Autodesk Fusion 360 part; units mm, degrees
(part 4 of 4)
  line L3219 (-15, -90.7321) -> (-14, -90.7321)
  line L3220 (-23, -90.7321) -> (-22.5, -89.866)
  line L3221 (-27, -89) -> (-27.5, -89.866)
  line L3222 (-23, -89) -> (-24, -89)
  line L3223 (-42, -90.7321) -> (-41, -90.7321)
  line L3224 (-48, -90.7321) -> (-47, -90.7321)
  line L3225 (-27, -90.7321) -> (-26, -90.7321)
  line L3226 (-47, -90.7321) -> (-46.5, -89.866)
  line L3227 (-47, -89) -> (-48, -89)
  line L3228 (-26, -89) -> (-27, -89)
  line L3229 (-48, -89) -> (-48.5, -89.866)
  line L3230 (-27.5, -89.866) -> (-27, -90.7321)
  line L3231 (-21, -89) -> (-21.5, -89.866)
  line L3232 (-19.5, -89.866) -> (-20, -89)
  line L3233 (-22.5, -89.866) -> (-23, -89)
  line L3234 (-26, -90.7321) -> (-25.5, -89.866)
  line L3235 (-25.5, -89.866) -> (-26, -89)
  line L3236 (-24, -89) -> (-24.5, -89.866)
  line L3237 (-45.5, -89.866) -> (-45, -90.7321)
  line L3238 (-21, -90.7321) -> (-20, -90.7321)
  line L3239 (-24.5, -89.866) -> (-24, -90.7321)
  line L3240 (-48.5, -89.866) -> (-48, -90.7321)
  line L3241 (-20, -90.7321) -> (-19.5, -89.866)
  line L3242 (-24, -90.7321) -> (-23, -90.7321)
  line L3243 (-14, -89) -> (-15, -89)
  point P0 (-68.5, -11.866)
  point P1 (-62.5, -11.866)
  point P2 (-56.5, -11.866)
  point P3 (-50.5, -11.866)
  point P4 (-44.5, -11.866)
  point P5 (-38.5, -11.866)
  point P6 (-32.5, -11.866)
  point P7 (-26.5, -11.866)
  point P8 (-20.5, -11.866)
  point P9 (-14.5, -11.866)
  point P10 (-68.5, -14.866)
  point P11 (-62.5, -14.866)
  point P12 (-56.5, -14.866)
  point P13 (-50.5, -14.866)
  point P14 (-44.5, -14.866)
  point P15 (-38.5, -14.866)
  point P16 (-26.5, -14.866)
  point P17 (-32.5, -14.866)
  point P18 (-20.5, -14.866)
  point P19 (-14.5, -14.866)
  point P20 (-68.5, -17.866)
  point P21 (-62.5, -20.866)
  point P22 (-44.5, -20.866)
  point P23 (-56.5, -20.866)
  point P24 (-50.5, -20.866)
  point P25 (-20.5, -20.866)
  point P26 (-32.5, -20.866)
  point P27 (-38.5, -20.866)
  point P28 (-26.5, -20.866)
  point P29 (-14.5, -20.866)
  point P30 (-62.5, -17.866)
  point P31 (-56.5, -17.866)
  point P32 (-50.5, -17.866)
  point P33 (-44.5, -17.866)
  point P34 (-38.5, -17.866)
  point P35 (-26.5, -17.866)
  point P36 (-32.5, -17.866)
  point P37 (-20.5, -17.866)
  point P38 (-14.5, -17.866)
  point P39 (-68.5, -20.866)
  point P40 (-68.5, -23.866)
  point P41 (-62.5, -26.866)
  point P42 (-44.5, -26.866)
  point P43 (-56.5, -26.866)
  point P44 (-50.5, -26.866)
  point P45 (-20.5, -26.866)
  point P46 (-32.5, -26.866)
  point P47 (-38.5, -26.866)
  point P48 (-26.5, -26.866)
  point P49 (-14.5, -26.866)
  point P50 (-44.5, -32.866)
  point P51 (-62.5, -32.866)
  point P52 (-56.5, -32.866)
  point P53 (-68.5, -29.866)
  point P54 (-50.5, -32.866)
  point P55 (-32.5, -32.866)
  point P56 (-38.5, -32.866)
  point P57 (-20.5, -32.866)
  point P58 (-26.5, -32.866)
  point P59 (-14.5, -32.866)
  point P60 (-62.5, -29.866)
  point P61 (-56.5, -29.866)
  point P62 (-50.5, -29.866)
  point P63 (-44.5, -29.866)
  point P64 (-20.5, -29.866)
  point P65 (-26.5, -29.866)
  point P66 (-38.5, -29.866)
  point P67 (-32.5, -29.866)
  point P68 (-68.5, -32.866)
  point P69 (-14.5, -29.866)
  point P70 (-62.5, -23.866)
  point P71 (-56.5, -23.866)
  point P72 (-50.5, -23.866)
  point P73 (-44.5, -23.866)
  point P74 (-38.5, -23.866)
  point P75 (-26.5, -23.866)
  point P76 (-32.5, -23.866)
  point P77 (-20.5, -23.866)
  point P78 (-14.5, -23.866)
  point P79 (-68.5, -26.866)
  point P80 (-68.5, -35.866)
  point P81 (-62.5, -38.866)
  point P82 (-44.5, -38.866)
  point P83 (-56.5, -38.866)
  point P84 (-50.5, -38.866)
  point P85 (-20.5, -38.866)
  point P86 (-32.5, -38.866)
  point P87 (-38.5, -38.866)
  point P88 (-26.5, -38.866)
  point P89 (-14.5, -38.866)
  point P90 (-44.5, -44.866)
  point P91 (-62.5, -44.866)
  point P92 (-56.5, -44.866)
  point P93 (-68.5, -41.866)
  point P94 (-50.5, -44.866)
  point P95 (-32.5, -44.866)
  point P96 (-38.5, -44.866)
  point P97 (-20.5, -44.866)
  point P98 (-26.5, -44.866)
  point P99 (-14.5, -44.866)
  point P100 (-62.5, -41.866)
  point P101 (-56.5, -41.866)
  point P102 (-50.5, -41.866)
  point P103 (-44.5, -41.866)
  point P104 (-62.5, -53.866)
  point P105 (-14.5, -56.866)
  point P106 (-56.5, -53.866)
  point P107 (-50.5, -53.866)
  point P108 (-26.5, -53.866)
  point P109 (-44.5, -53.866)
  point P110 (-38.5, -53.866)
  point P111 (-20.5, -53.866)
  point P112 (-32.5, -53.866)
  point P113 (-68.5, -56.866)
  point P114 (-62.5, -47.866)
  point P115 (-14.5, -53.866)
  point P116 (-56.5, -47.866)
  point P117 (-50.5, -47.866)
  point P118 (-26.5, -47.866)
  point P119 (-38.5, -47.866)
  point P120 (-44.5, -47.866)
  point P121 (-20.5, -47.866)
  point P122 (-32.5, -47.866)
  point P123 (-14.5, -47.866)
  point P124 (-68.5, -50.866)
  point P125 (-20.5, -41.866)
  point P126 (-26.5, -41.866)
  point P127 (-38.5, -41.866)
  point P128 (-32.5, -41.866)
  point P129 (-68.5, -44.866)
  point P130 (-14.5, -41.866)
  point P131 (-68.5, -47.866)
  point P132 (-62.5, -50.866)
  point P133 (-50.5, -50.866)
  point P134 (-44.5, -50.866)
  point P135 (-56.5, -50.866)
  point P136 (-32.5, -50.866)
  point P137 (-20.5, -50.866)
  point P138 (-26.5, -50.866)
  point P139 (-38.5, -50.866)
  point P140 (-14.5, -50.866)
  point P141 (-44.5, -56.866)
  point P142 (-68.5, -53.866)
  point P143 (-50.5, -56.866)
  point P144 (-62.5, -56.866)
  point P145 (-56.5, -56.866)
  point P146 (-32.5, -56.866)
  point P147 (-38.5, -56.866)
  point P148 (-26.5, -56.866)
  point P149 (-20.5, -56.866)
  point P150 (-62.5, -35.866)
  point P151 (-56.5, -35.866)
  point P152 (-50.5, -35.866)
  point P153 (-44.5, -35.866)
  point P154 (-38.5, -35.866)
  point P155 (-26.5, -35.866)
  point P156 (-32.5, -35.866)
  point P157 (-20.5, -35.866)
  point P158 (-14.5, -35.866)
  point P159 (-68.5, -38.866)
  point P160 (-14.5, -59.866)
  point P161 (-68.5, -62.866)
  point P162 (-68.5, -65.866)
  point P163 (-62.5, -68.866)
  point P164 (-50.5, -68.866)
  point P165 (-44.5, -68.866)
  point P166 (-32.5, -68.866)
  point P167 (-56.5, -68.866)
  point P168 (-20.5, -68.866)
  point P169 (-26.5, -68.866)
  point P170 (-38.5, -68.866)
  point P171 (-68.5, -71.866)
  point P172 (-44.5, -74.866)
  point P173 (-50.5, -74.866)
  point P174 (-14.5, -68.866)
  point P175 (-62.5, -74.866)
  point P176 (-56.5, -74.866)
  point P177 (-32.5, -74.866)
  point P178 (-38.5, -74.866)
  point P179 (-26.5, -74.866)
  point P180 (-20.5, -74.866)
  point P181 (-56.5, -71.866)
  point P182 (-14.5, -74.866)
  point P183 (-50.5, -71.866)
  point P184 (-44.5, -71.866)
  point P185 (-26.5, -71.866)
  point P186 (-20.5, -71.866)
  point P187 (-38.5, -71.866)
  point P188 (-32.5, -71.866)
  point P189 (-68.5, -74.866)
  point P190 (-62.5, -65.866)
  point P191 (-50.5, -65.866)
  point P192 (-56.5, -65.866)
  point P193 (-14.5, -71.866)
  point P194 (-26.5, -65.866)
  point P195 (-38.5, -65.866)
  point P196 (-44.5, -65.866)
  point P197 (-20.5, -65.866)
  point P198 (-32.5, -65.866)
  point P199 (-14.5, -65.866)
  point P200 (-38.5, -59.866)
  point P201 (-20.5, -59.866)
  point P202 (-68.5, -68.866)
  point P203 (-26.5, -59.866)
  point P204 (-32.5, -59.866)
  point P205 (-50.5, -59.866)
  point P206 (-44.5, -59.866)
  point P207 (-62.5, -71.866)
  point P208 (-44.5, -62.866)
  point P209 (-62.5, -62.866)
  point P210 (-68.5, -59.866)
  point P211 (-50.5, -62.866)
  point P212 (-56.5, -62.866)
  point P213 (-38.5, -62.866)
  point P214 (-32.5, -62.866)
  point P215 (-20.5, -62.866)
  point P216 (-62.5, -59.866)
  point P217 (-26.5, -62.866)
  point P218 (-14.5, -62.866)
  point P219 (-56.5, -59.866)
  point P220 (-50.5, -80.866)
  point P221 (-68.5, -77.866)
  point P222 (-44.5, -80.866)
  point P223 (-62.5, -80.866)
  point P224 (-56.5, -80.866)
  point P225 (-32.5, -80.866)
  point P226 (-38.5, -80.866)
  point P227 (-14.5, -80.866)
  point P228 (-26.5, -80.866)
  point P229 (-20.5, -80.866)
  point P230 (-56.5, -77.866)
  point P231 (-50.5, -77.866)
  point P232 (-26.5, -77.866)
  point P233 (-44.5, -77.866)
  point P234 (-20.5, -77.866)
  point P235 (-38.5, -77.866)
  point P236 (-32.5, -77.866)
  point P237 (-68.5, -80.866)
  point P238 (-14.5, -77.866)
  point P239 (-62.5, -77.866)
  point P240 (-56.5, -86.866)
  point P241 (-62.5, -86.866)
  point P242 (-32.5, -86.866)
  point P243 (-50.5, -86.866)
  point P244 (-68.5, -83.866)
  point P245 (-44.5, -86.866)
  point P246 (-38.5, -86.866)
  point P247 (-26.5, -86.866)
  point P248 (-20.5, -86.866)
  point P249 (-14.5, -86.866)
  point P250 (-56.5, -83.866)
  point P251 (-26.5, -83.866)
  point P252 (-44.5, -83.866)
  point P253 (-50.5, -83.866)
  point P254 (-20.5, -83.866)
  point P255 (-38.5, -83.866)
  point P256 (-14.5, -83.866)
  point P257 (-32.5, -83.866)
  point P258 (-68.5, -86.866)
  point P259 (-62.5, -83.866)
  point P260 (-68.5, -89.866)
  point P261 (-62.5, -89.866)
  point P262 (-32.5, -89.866)
  point P263 (-56.5, -89.866)
  point P264 (-44.5, -89.866)
  point P265 (-38.5, -89.866)
  point P266 (-26.5, -89.866)
  point P267 (-20.5, -89.866)
  point P268 (-50.5, -89.866)
  point P269 (-14.5, -89.866)
extrude "Extrude11" cut sketch "Sketch7" against normal blind 5 contours L3 L3154 L3157 L3162 | L3 L3149 L3154 L3162 L3164 L3167 | L3 L3159 L3169 L3219 | L3 L3153 L3159 L3163 L3169 L3243 | L3 L3133 L3134 L3141 L3144 L3204 | L3 L3133 L3141 L3202 | L3 L3151 L3161 L3166 | L3 L3148 L3151 L3155 L3158 L3161 | L3 L3138 L3143 L3196 L3197 L3198 | L3 L3135 L3138 L3197 | L3 L3217 L3238 L3241 | L3 L3217 L3218 L3231 L3232 L3241 | L3 L3128 L3207 L3209 L3212 L3213 | L3 L3128 L3207 L3215 | L3 L3220 L3239 L3242 | L3 L3220 L3222 L3233 L3236 L3239 | L3 L3124 L3130 L3210 L3214 L3216 | L3 L3124 L3126 L3130 | L3 L3225 L3230 L3234 | L3 L3221 L3228 L3230 L3234 L3235 | L3 L3125 L3129 L3206 L3208 L3211 | L3 L3125 L3129 L3139 | L3 L3171 L3179 L3181 | L3 L3175 L3179 L3181 L3187 L3194 | L3 L3127 L3136 L3142 L3200 L3205 | L3 L3136 L3142 L3203 | L3 L3178 L3190 L3192 | L3 L3174 L3177 L3184 L3190 L3192 | L3 L3131 L3137 L3140 L3195 L3201 | L3 L3132 L3140 L3201 | L3 L3176 L3180 L3193 | L3 L3173 L3176 L3182 L3185 L3193 | L3 L3199 L3226 L3227 L3229 L3240 | L3 L3224 L3226 L3240 | L3 L3170 L3183 L3186 | L3 L3170 L3172 L3183 L3188 L3189 | L3 L3147 L3150 L3168 L3191 L3237 | L3 L3165 L3168 L3237 | L3 L3152 L3160 L3223 | L3 L3145 L3146 L3152 L3156 L3160 | L4 L5 L6 L7 L8 L9 | L10 L11 L12 L13 L14 L15 | L16 L17 L22 L24 L26 L27 | L18 L19 L20 L21 L23 L25 | L28 L29 L36 L38 L41 L48 | L30 L31 L37 L39 L50 L51 | L32 L34 L35 L42 L46 L47 | L33 L40 L43 L44 L45 L49 | L52 L54 L57 L94 L96 L98 | L53 L63 L72 L85 L95 L99 | L55 L60 L64 L70 L71 L73 | L56 L62 L66 L90 L92 L93 | L58 L76 L77 L79 L80 L91 | L59 L75 L82 L84 L88 L89 | L61 L65 L67 L68 L69 L97 | L74 L78 L81 L83 L86 L87 | L100 L102 L103 L106 L107 L111 | L101 L104 L105 L108 L109 L110 | L112 L113 L114 L117 L120 L123 | L115 L116 L118 L119 L121 L122 | L124 L137 L138 L140 L183 L238 | L125 L200 L202 L204 L213 L218 | L126 L134 L214 L217 L221 L225 | L127 L128 L130 L192 L216 L235 | L129 L195 L209 L211 L230 L234 | L131 L190 L197 L198 L212 L227 | L132 L136 L193 L206 L224 L226 | L133 L187 L203 L205 L219 L222 | L135 L188 L189 L208 L223 L233 | L139 L142 L144 L177 L180 L241 | L141 L149 L151 L174 L182 L185 | L143 L145 L172 L184 L242 L243 | L146 L154 L157 L162 L167 L170 | L147 L148 L150 L153 L161 L169 | L152 L155 L173 L179 L181 L237 | L156 L158 L163 L164 L166 L231 | L159 L160 L165 L168 L171 L228 | L175 L176 L178 L186 L239 L240 | L191 L194 L196 L199 L207 L229 | L201 L210 L215 L220 L232 L236 | L244 L246 L250 L426 L428 L439 | L245 L247 L254 L262 L315 L415 | L248 L259 L261 L413 L417 L421 | L249 L251 L252 L255 L311 L414 | L253 L307 L308 L416 L423 L424 | L256 L257 L429 L430 L435 L436 | L258 L304 L419 L422 L431 L438 | L260 L316 L412 L432 L433 L437 | L263 L265 L280 L286 L295 L296 | L264 L276 L302 L447 L474 L476 | L266 L272 L275 L277 L288 L298 | L267 L273 L440 L443 L446 L483 | L268 L283 L297 L442 L467 L473 | L269 L270 L282 L287 L293 L303 | L271 L289 L479 L480 L481 L482 | L274 L279 L291 L292 L299 L301 | L278 L281 L284 L300 L441 L475 | L285 L290 L294 L444 L456 L478 | L305 L310 L313 L314 L420 L427 | L306 L309 L312 L418 L425 L434 | L317 L321 L326 L331 L397 L398 | L318 L319 L330 L391 L392 L406 | L320 L375 L377 L384 L388 L410 | L322 L329 L332 L389 L395 L407 | L323 L327 L328 L376 L385 L396 | L324 L325 L374 L386 L387 L390 | L333 L343 L352 L358 L365 L470 | L334 L344 L369 L383 L394 L399 | L335 L348 L351 L357 L381 L411 | L336 L337 L342 L359 L380 L393 | L338 L347 L368 L382 L401 L408 | L339 L346 L355 L370 L371 L378 | L340 L350 L353 L366 L372 L404 | L341 L373 L445 L448 L449 L477 | L345 L356 L361 L364 L465 L468 | L349 L367 L402 L403 L405 L472 | L354 L362 L363 L379 L400 L409 | L360 L450 L451 L454 L461 L469 | L452 L459 L460 L462 L463 L471 | L453 L455 L457 L458 L464 L466 | L484 L497 L502 L503 L953 L955 | L485 L489 L490 L494 L496 L505 | L486 L493 L499 L500 L508 L952 | L487 L491 L498 L504 L507 L960 | L488 L495 L506 L961 L962 L963 | L492 L501 L951 L957 L958 L959 | L509 L831 L833 L836 L861 L864 | L510 L512 L767 L773 L775 L863 | L511 L513 L772 L832 L837 L956 | L514 L515 L517 L768 L774 L835 | L516 L765 L766 L769 L770 L954 | L518 L771 L830 L834 L860 L862 | L519 L526 L540 L554 L561 L704 | L520 L528 L578 L589 L590 L600 | L521 L531 L538 L545 L547 L568 | L522 L539 L552 L574 L579 L594 | L523 L542 L543 L548 L690 L694 | L524 L534 L553 L557 L569 L570 | L525 L527 L537 L549 L551 L563 | L529 L530 L535 L550 L556 L572 | L532 L533 L677 L682 L696 L699 | L536 L571 L585 L586 L587 L593 | L541 L546 L678 L688 L697 L700 | L544 L558 L559 L562 L675 L684 | L555 L564 L575 L576 L601 L602 | L560 L673 L681 L691 L698 L702 | L565 L685 L693 L695 L703 L706 | L566 L591 L592 L808 L816 L820 | L567 L573 L793 L809 L818 L825 | L577 L595 L599 L819 L826 L827 | L580 L596 L790 L794 L798 L807 | L581 L604 L792 L804 L805 L828 | L582 L605 L800 L803 L821 L829 | L583 L796 L813 L815 L817 L823 | L584 L588 L598 L802 L812 L814 | L597 L603 L795 L799 L806 L810 | L606 L635 L662 L663 L668 L672 | L607 L617 L634 L648 L667 L670 | L608 L679 L721 L730 L735 L742 | L609 L613 L615 L618 L641 L652 | L610 L612 L627 L644 L650 L657 | L611 L616 L623 L640 L727 L736 | L614 L633 L649 L651 L669 L671 | L619 L626 L716 L717 L731 L741 | L620 L624 L625 L653 L654 L661 | L621 L630 L631 L642 L665 L666 | L622 L637 L639 L647 L659 L660 | L628 L636 L646 L655 L656 L664 | L629 L632 L638 L643 L645 L658 | L674 L689 L701 L733 L737 L738 | L676 L680 L686 L687 L692 L705 | L683 L708 L723 L725 L728 L734 | L707 L711 L712 L713 L722 L724 | L709 L710 L718 L719 L720 L729 | L714 L715 L726 L732 L739 L740 | L743 L745 L762 L873 L875 L914 | L744 L748 L751 L753 L760 L878 | L746 L752 L754 L755 L764 L882 | L747 L750 L759 L763 L879 L880 | L749 L756 L757 L758 L877 L883 | L761 L874 L876 L881 L884 L885 | L776 L781 L783 L789 L845 L856 | L777 L787 L838 L849 L857 L858 | L778 L779 L786 L840 L848 L853 | L780 L784 L839 L844 L851 L855 | L782 L785 L788 L841 L852 L854 | L791 L797 L801 L811 L822 L824 | L842 L843 L846 L847 L850 L859 | L865 L866 L871 L918 L925 L949 | L867 L869 L894 L898 L904 L938 | L868 L888 L902 L910 L912 L923 | L870 L908 L909 L913 L934 L942 | L872 L886 L903 L919 L922 L926 | L887 L890 L899 L900 L901 L916 | L889 L915 L930 L944 L946 L947 | L891 L897 L921 L931 L940 L950 | L892 L924 L928 L936 L943 L945 | L893 L895 L905 L920 L935 L939 | L896 L907 L911 L917 L937 L941 | L906 L927 L929 L932 L933 L948 | L964 L978 L1056 L1066 L1714 L1724 | L965 L997 L999 L1005 L1719 L1725 | L966 L967 L972 L990 L1004 L1734 | L968 L998 L1007 L1040 L1063 L1732 | L969 L995 L1002 L1006 L1047 L1740 | L970 L979 L985 L1001 L1043 L1074 | L971 L975 L980 L1721 L1723 L1730 | L973 L981 L983 L984 L989 L992 | L974 L982 L991 L1713 L1715 L1735 | L976 L1000 L1044 L1048 L1050 L1731 | L977 L987 L988 L1736 L1737 L1738 | L986 L993 L994 L996 L1003 L1712 | L1008 L1012 L1016 L1070 L1781 L1792 | L1009 L1013 L1017 L1026 L1029 L1090 | L1010 L1019 L1028 L1079 L1083 L1085 | L1011 L1021 L1023 L1031 L1062 L1089 | L1014 L1015 L1024 L1071 L1076 L1086 | L1018 L1381 L1405 L1410 L1779 L1914 | L1020 L1776 L1778 L1793 L1798 L1804 | L1022 L1058 L1068 L1077 L1084 L1091 | L1025 L1033 L1037 L1059 L1780 L1797 | L1027 L1032 L1036 L1054 L1787 L1795 | L1030 L1061 L1069 L1081 L1087 L1088 | L1034 L1035 L1064 L1067 L1072 L1080 | L1038 L1039 L1046 L1052 L1075 L1078 | L1041 L1042 L1045 L1053 L1057 L1065 | L1049 L1051 L1055 L1060 L1073 L1082 | L1092 L1106 L1116 L1119 L1624 L1625 | L1093 L1095 L1109 L1110 L1629 L1649 | L1094 L1103 L1120 L1135 L1136 L1655 | L1096 L1097 L1125 L1129 L1131 L1636 | L1098 L1122 L1677 L1812 L1818 L1838 | L1099 L1651 L1675 L1680 L1816 L1831 | L1100 L1114 L1657 L1659 L1661 L1690 | L1101 L1126 L1138 L1660 L1664 L1689 | L1102 L1112 L1113 L1128 L1623 L1694 | L1104 L1672 L1678 L1692 L1829 L1851 | L1105 L1665 L1666 L1667 L1691 L1693 | L1107 L1142 L1152 L1616 L1646 L1648 | L1108 L1123 L1124 L1130 L1132 L1634 | L1111 L1153 L1569 L1627 L1641 L1647 | L1115 L1117 L1121 L1622 L1628 L1638 | L1118 L1127 L1133 L1134 L1615 L1626 | L1137 L1618 L1630 L1642 L1643 L1644 | L1139 L1140 L1570 L1590 L1607 L1609 | L1141 L1147 L1171 L1189 L1190 L1704 | L1143 L1162 L1586 L1600 L1603 L1613 | L1144 L1149 L1154 L1158 L1163 L1611 | L1145 L1150 L1175 L1178 L1181 L1697 | L1146 L1608 L1621 L1633 L1635 L1637 | L1148 L1157 L1160 L1165 L1166 L1606 | L1151 L1156 L1167 L1173 L1182 L1574 | L1155 L1177 L1179 L1421 L1426 L1707 | L1159 L1161 L1164 L1573 L1610 L1612 | L1168 L1170 L1174 L1176 L1695 L1764 | L1169 L1184 L1185 L1593 L1595 L1602 | L1172 L1180 L1428 L1699 L1766 L1768 | L1183 L1187 L1188 L1696 L1703 L1767 | L1186 L1418 L1427 L1706 L1717 L1765 | L1191 L1742 L1751 L1756 L1762 L1808 | L1192 L1194 L1196 L1198 L1837 L1846 | L1193 L1197 L1200 L1204 L1747 L1760 | L1195 L1202 L1211 L1219 L1819 L1849 | L1199 L1218 L1811 L1815 L1824 L1841 | L1201 L1208 L1212 L1749 L1755 L1761 | L1203 L1206 L1753 L1757 L1758 L1807 | L1205 L1210 L1215 L1217 L1839 L1847 | L1207 L1216 L1743 L1748 L1752 L1754 | L1209 L1822 L1832 L1840 L1842 L1845 | L1213 L1214 L1825 L1843 L1850 L1853 | L1220 L1224 L1262 L1275 L1295 L1296 | L1221 L1260 L1269 L1272 L1293 L1314 | L1222 L1249 L1279 L1280 L1294 L1502 | L1223 L1231 L1281 L1298 L1509 L1527 | L1225 L1273 L1282 L1288 L1516 L1541 | L1226 L1263 L1265 L1289 L1300 L1534 | L1227 L1242 L1245 L1255 L1256 L1285 | L1228 L1248 L1310 L1321 L1325 L1532 | L1229 L1236 L1243 L1286 L1311 L1317 | L1230 L1241 L1254 L1270 L1292 L1526 | L1232 L1246 L1274 L1287 L1290 L1506 | L1233 L1240 L1251 L1253 L1539 L1540 | L1234 L1244 L1258 L1283 L1291 L1316 | L1235 L1250 L1259 L1261 L1266 L1276 | L1237 L1257 L1268 L1320 L1336 L1504 | L1238 L1252 L1267 L1297 L1522 L1531 | L1239 L1318 L1332 L1342 L1346 L1347 | L1247 L1308 L1309 L1315 L1326 L1329 | L1264 L1271 L1278 L1299 L1305 L1306 | L1277 L1284 L1313 L1338 L1341 L1343 | L1301 L1327 L1353 L1435 L1438 L1455 | L1302 L1359 L1362 L1366 L1368 L1451 | L1303 L1304 L1340 L1344 L1367 L1372 | L1307 L1337 L1349 L1364 L1450 L1462 | L1312 L1322 L1323 L1330 L1331 L1335 | L1319 L1324 L1333 L1339 L1348 L1373 | L1328 L1334 L1352 L1360 L1361 L1371 | L1345 L1356 L1369 L1432 L1440 L1463 | L1350 L1354 L1355 L1363 L1444 L1466 | L1351 L1358 L1365 L1436 L1447 L1467 | L1357 L1437 L1458 L1460 L1461 L1468 | L1370 L1434 L1439 L1445 L1453 L1454 | L1374 L1376 L1441 L1456 L1464 L1465 | L1375 L1443 L1448 L1452 L1457 L1459 | L1377 L1379 L1400 L1414 L1788 L1796 | L1378 L1382 L1383 L1384 L1413 L1900 | L1380 L1392 L1401 L1407 L1412 L1901 | L1385 L1398 L1406 L1905 L1906 L1918 | L1386 L1391 L1393 L1395 L1404 L1416 | L1387 L1397 L1408 L1409 L1904 L1921 | L1388 L1389 L1415 L1899 L1919 L1922 | L1390 L1402 L1783 L1791 L1794 L1803 | L1394 L1396 L1782 L1790 L1800 L1801 | L1399 L1770 L1771 L1775 L1786 L1805 | L1403 L1411 L1769 L1773 L1774 L1785 | L1417 L1705 L1710 L1716 L1733 L1741 | L1419 L1422 L1700 L1709 L1711 L1729 | L1420 L1429 L1430 L1718 L1722 L1763 | L1423 L1698 L1701 L1720 L1726 L1739 | L1424 L1425 L1702 L1708 L1727 L1728 | L1431 L1446 L1477 L1484 L1493 L1498 | L1433 L1479 L1488 L1490 L1497 L1500 | L1442 L1496 L1866 L1879 L1885 L1888 | L1449 L1474 L1476 L1478 L1483 L1494 | L1469 L1482 L1865 L1874 L1882 L1913 | L1470 L1475 L1486 L1495 L1856 L1890 | L1471 L1481 L1860 L1870 L1896 L1911 | L1472 L1491 L1871 L1883 L1891 L1909 | L1473 L1489 L1855 L1863 L1881 L1892 | L1480 L1487 L1861 L1862 L1895 L1923 | L1485 L1499 L1869 L1884 L1886 L1887 | L1492 L1872 L1878 L1889 L1903 L1908 | L1501 L1517 L1524 L1525 L1549 L1554 | L1503 L1520 L1542 L1557 L1562 L1567 | L1505 L1529 L1536 L1538 L1558 L1561 | L1507 L1530 L1537 L1544 L1547 L1551 | L1508 L1533 L1546 L1552 L1564 L1565 | L1510 L1515 L1523 L1555 L1560 L1563 | L1511 L1512 L1513 L1535 L1545 L1566 | L1514 L1521 L1543 L1548 L1550 L1553 | L1518 L1519 L1528 L1556 L1559 L1568 | L1571 L1585 L1587 L1591 L1597 L1598 | L1572 L1575 L1577 L1579 L1631 L1650 | L1576 L1580 L1588 L1596 L1619 L1639 | L1578 L1581 L1584 L1589 L1592 L1640 | L1582 L1583 L1599 L1604 L1605 L1614 | L1594 L1601 L1617 L1620 L1632 L1645 | L1652 L1653 L1683 L1684 L1813 L1833 | L1654 L1676 L1817 L1823 L1827 L1835 | L1656 L1668 L1674 L1681 L1685 L1810 | L1658 L1673 L1821 L1826 L1834 L1852 | L1662 L1679 L1687 L1688 L1814 L1836 | L1663 L1820 L1828 L1830 L1844 L1848 | L1669 L1670 L1671 L1682 L1686 L1806 | L1744 L1745 L1746 L1750 L1759 L1809 | L1772 L1777 L1784 L1789 L1799 L1802 | L1854 L1864 L1867 L1868 L1880 L1897 | L1857 L1873 L1875 L1877 L1893 L1916 | L1858 L1859 L1876 L1894 L1910 L1912 | L1898 L1902 L1907 L1915 L1917 L1920 | L1924 L2272 L2275 L2634 L2640 L2642 | L1925 L1927 L2261 L2263 L2264 L2635 | L1926 L2266 L2268 L2270 L2638 L2639 | L1928 L1946 L1947 L1948 L1951 L1958 | L1929 L1935 L1939 L1944 L1952 L1961 | L1930 L1940 L1943 L2021 L2024 L2034 | L1931 L1942 L1950 L1955 L2014 L2036 | L1932 L1933 L1937 L2018 L2027 L2039 | L1934 L1949 L1954 L1964 L2022 L2038 | L1936 L1945 L1960 L1962 L1965 L1997 | L1938 L2011 L2013 L2019 L2031 L2032 | L1941 L2012 L2015 L2020 L2023 L2037 | L1953 L1956 L1957 L1959 L1963 L2001 | L1966 L1977 L1988 L1989 L2250 L2252 | L1967 L1980 L1984 L1986 L1995 L2002 | L1968 L2208 L2215 L2236 L2240 L2258 | L1969 L1970 L1976 L1982 L1985 L1987 | L1971 L1972 L1978 L1979 L1983 L1996 | L1973 L1991 L2511 L2516 L2577 L2598 | L1974 L1999 L2509 L2536 L2610 L2617 | L1975 L1981 L2552 L2558 L2597 L2614 | L1990 L2227 L2246 L2256 L2537 L2540 | L1992 L2204 L2211 L2248 L2251 L2253 | L1993 L1998 L2000 L2003 L2005 L2008 | L1994 L2004 L2006 L2007 L2009 L2010 | L2016 L2017 L2025 L2026 L2030 L2288 | L2028 L2029 L2033 L2035 L2279 L2283 | L2040 L2055 L2060 L2081 L2414 L2423 | L2041 L2045 L2048 L2062 L2419 L2620 | L2042 L2075 L2083 L2088 L2091 L2097 | L2043 L2046 L2047 L2054 L2066 L2068 | L2044 L2049 L2073 L2079 L2082 L2090 | L2050 L2052 L2056 L2059 L2412 L2484 | L2051 L2053 L2065 L2074 L2471 L2488 | L2057 L2061 L2063 L2086 L2434 L2459 | L2058 L2064 L2069 L2092 L2448 L2474 | L2067 L2071 L2084 L2085 L2094 L2099 | L2070 L2076 L2080 L2089 L2093 L2096 | L2072 L2077 L2078 L2087 L2095 L2098 | L2100 L2102 L2129 L2137 L2148 L2150 | L2101 L2104 L2115 L2149 L2151 L2154 | L2103 L2124 L2203 L2302 L2371 L2381 | L2105 L2110 L2118 L2142 L2144 L2153 | L2106 L2117 L2125 L2146 L2157 L2608 | L2107 L2120 L2122 L2133 L2143 L2147 | L2108 L2109 L2113 L2119 L2138 L2145 | L2111 L2127 L2317 L2332 L2384 L2397 | L2112 L2136 L2305 L2308 L2375 L2377 | L2114 L2123 L2126 L2132 L2152 L2156 | L2116 L2562 L2586 L2591 L2602 L2609 | L2121 L2588 L2596 L2605 L2613 L2615 | L2128 L2141 L2160 L2579 L2601 L2604 | L2130 L2134 L2139 L2140 L2155 L2158 | L2131 L2183 L2361 L2390 L2392 L2394 | L2135 L2161 L2165 L2166 L2184 L2191 | L2159 L2169 L2172 L2173 L2175 L2193 | L2162 L2170 L2350 L2354 L2383 L2395 | L2163 L2171 L2178 L2185 L2187 L2188 | L2164 L2174 L2176 L2180 L2182 L2186 | L2167 L2168 L2179 L2181 L2189 L2192 | L2177 L2190 L2337 L2352 L2368 L2370 | L2194 L2198 L2201 L2310 L2318 L2322 | L2195 L2197 L2298 L2301 L2309 L2323 | L2196 L2328 L2429 L2437 L2490 L2493 | L2199 L2303 L2306 L2311 L2325 L2330 | L2200 L2202 L2304 L2314 L2335 L2351 | L2205 L2206 L2574 L2590 L2594 L2599 | L2207 L2213 L2218 L2232 L2245 L2254 | L2209 L2231 L2521 L2544 L2548 L2553 | L2210 L2212 L2220 L2229 L2239 L2259 | L2214 L2223 L2238 L2241 L2244 L2255 | L2216 L2221 L2224 L2237 L2249 L2257 | L2217 L2507 L2512 L2513 L2534 L2547 | L2219 L2242 L2243 L2501 L2522 L2533 | L2222 L2228 L2518 L2542 L2546 L2554 | L2225 L2226 L2235 L2532 L2535 L2556 | L2230 L2233 L2524 L2569 L2593 L2611 | L2234 L2247 L2566 L2578 L2595 L2606 | L2260 L2267 L2273 L2274 L2637 L2641 | L2262 L2269 L2271 L2294 L2297 L2630 | L2265 L2286 L2290 L2627 L2636 L2643 | L2276 L2280 L2281 L2282 L2287 L2632 | L2277 L2284 L2291 L2295 L2623 L2628 | L2278 L2296 L2624 L2626 L2629 L2631 | L2285 L2289 L2292 L2293 L2625 L2633 | L2299 L2300 L2316 L2319 L2320 L2329 | L2307 L2362 L2420 L2440 L2476 L2494 | L2312 L2313 L2315 L2321 L2326 L2331 | L2324 L2327 L2402 L2411 L2426 L2497 | L2333 L2334 L2339 L2340 L2345 L2353 | L2336 L2338 L2355 L2374 L2380 L2388 | L2341 L2343 L2344 L2356 L2360 L2364 | L2342 L2346 L2359 L2366 L2369 L2387 | L2347 L2363 L2365 L2367 L2389 L2391 | L2348 L2349 L2433 L2457 L2485 L2489 | L2357 L2358 L2407 L2415 L2452 L2479 | L2372 L2378 L2379 L2385 L2393 L2396 | L2373 L2376 L2465 L2480 L2487 L2492 | L2382 L2398 L2399 L2403 L2428 L2432 | L2386 L2401 L2405 L2430 L2438 L2441 | L2400 L2404 L2406 L2431 L2435 L2436 | L2408 L2413 L2482 L2495 L2498 L2499 | L2409 L2417 L2425 L2619 L2621 L2622 | L2410 L2416 L2421 L2466 L2483 L2486 | L2418 L2422 L2424 L2444 L2464 L2478 | L2427 L2439 L2445 L2454 L2458 L2473 | L2442 L2447 L2455 L2468 L2469 L2477 | L2443 L2453 L2456 L2462 L2467 L2472 | L2446 L2450 L2460 L2461 L2470 L2475 | L2449 L2451 L2463 L2481 L2491 L2496 | L2500 L2503 L2573 L2581 L2582 L2583 | L2502 L2505 L2526 L2529 L2567 L2584 | L2504 L2517 L2519 L2520 L2527 L2565 | L2506 L2559 L2563 L2570 L2585 L2589 | L2508 L2514 L2525 L2530 L2545 L2549 | L2510 L2515 L2523 L2539 L2543 L2550 | L2528 L2564 L2568 L2575 L2580 L2587 | L2531 L2538 L2541 L2551 L2555 L2557 | L2560 L2561 L2571 L2592 L2603 L2616 | L2572 L2576 L2600 L2607 L2612 L2618 | L2644 L2645 L2683 L2684 L2685 L2702 | L2646 L2658 L2695 L2698 L2699 L2700 | L2647 L2649 L2682 L2692 L2838 L2875 | L2648 L2665 L2827 L2831 L2840 L2860 | L2650 L2664 L2688 L2691 L2854 L2857 | L2651 L2668 L2676 L2837 L2852 L2873 | L2652 L2653 L2667 L2678 L2686 L2690 | L2654 L2689 L2693 L2828 L2841 L2851 | L2655 L2671 L2674 L2679 L2687 L2872 | L2656 L2660 L2666 L2673 L2675 L2694 | L2657 L2669 L2672 L2681 L2849 L2874 | L2659 L2661 L2662 L2663 L2855 L2871 | L2670 L2680 L2696 L2697 L2703 L2706 | L2677 L2701 L2704 L2705 L2707 L2850 | L2708 L2775 L2795 L2797 L2876 L2881 | L2709 L2764 L2768 L2773 L2776 L2779 | L2710 L2772 L2799 L2801 L2803 L2879 | L2711 L2760 L2761 L2762 L2767 L2769 | L2712 L2777 L2781 L2809 L2811 L2813 | L2713 L2717 L2723 L2725 L2729 L2731 | L2714 L2719 L2722 L2726 L2728 L2736 | L2715 L2720 L2721 L2730 L2734 L2735 | L2716 L2718 L2724 L2727 L2732 L2733 | L2737 L2738 L2754 L2756 L2757 L2771 | L2739 L2742 L2745 L2746 L2751 L2752 | L2740 L2744 L2748 L2749 L2750 L2759 | L2741 L2743 L2747 L2753 L2755 L2758 | L2763 L2765 L2807 L2810 L2877 L2878 | L2766 L2778 L2782 L2880 L2882 L2883 | L2770 L2774 L2785 L2786 L2812 L2814 | L2780 L2796 L2798 L2804 L2806 L2808 | L2783 L2793 L2794 L2800 L2802 L2805 | L2784 L2787 L2789 L2829 L2836 L2861 | L2788 L2816 L2821 L2825 L2834 L2856 | L2790 L2791 L2792 L2817 L2822 L2832 | L2815 L2818 L2819 L2823 L2826 L2830 | L2820 L2833 L2835 L2843 L2844 L2862 | L2824 L2839 L2846 L2853 L2867 L2868 | L2842 L2848 L2858 L2865 L2866 L2869 | L2845 L2847 L2859 L2863 L2864 L2870 | L2884 L2886 L2889 L2893 L2920 L2946 | L2885 L2887 L2894 L2909 L2922 L2936 | L2888 L2890 L2892 L2907 L2910 L2952 | L2891 L2895 L2908 L2937 L2941 L2942 | L2896 L2898 L2902 L2904 L2905 L2916 | L2897 L2899 L2901 L2906 L2917 L3113 | L2900 L2903 L2913 L2914 L3099 L3109 | L2911 L2912 L2915 L3094 L3095 L3100 | L2918 L2928 L3008 L3012 L3017 L3018 | L2919 L2955 L2958 L2962 L2974 L2987 | L2921 L2929 L2931 L2938 L2940 L2943 | L2923 L2925 L2930 L2934 L2935 L2947 | L2924 L2933 L3003 L3019 L3020 L3021 | L2926 L2950 L2951 L2954 L2967 L2992 | L2927 L2932 L2975 L2994 L3011 L3016 | L2939 L2944 L2949 L2956 L2957 L2983 | L2945 L2966 L2970 L2977 L2981 L3006 | L2948 L2953 L2998 L3002 L3013 L3014 | L2959 L2960 L2969 L2993 L2996 L2997 | L2961 L2963 L2980 L2988 L2995 L3007 | L2964 L2965 L2968 L2979 L2990 L2991 | L2971 L2973 L2999 L3000 L3009 L3015 | L2972 L2982 L2984 L2986 L2989 L3004 | L2976 L2978 L2985 L3001 L3005 L3010 | L3022 L3033 L3038 L3114 L3122 L3123 | L3023 L3025 L3029 L3047 L3049 L3057 | L3024 L3037 L3052 L3053 L3065 L3119 | L3026 L3027 L3028 L3048 L3117 L3121 | L3030 L3034 L3035 L3061 L3116 L3120 | L3031 L3039 L3063 L3067 L3080 L3082 | L3032 L3040 L3062 L3066 L3072 L3086 | L3036 L3043 L3046 L3054 L3115 L3118 | L3041 L3044 L3064 L3074 L3081 L3101 | L3042 L3045 L3055 L3084 L3088 L3106 | L3050 L3056 L3083 L3087 L3096 L3112 | L3051 L3058 L3070 L3073 L3075 L3079 | L3059 L3069 L3076 L3077 L3078 L3110 | L3060 L3068 L3071 L3085 L3090 L3107 | L3089 L3092 L3098 L3102 L3105 L3111 | L3091 L3093 L3097 L3103 L3104 L3108 bodies 3
sketch "Sketch8" plane through (0, 24, 0) normal (0, -1, 0) x (1, 0, 0)
  line L0 (60.6044, -92.1931) -> (18.6044, -92.1931)
  line L1 (18.6044, -92.1931) -> (18.6044, -7.1931)
  line L2 (18.6044, -7.1931) -> (60.6044, -7.1931)
  line L3 (60.6044, -7.1931) -> (60.6044, -92.1931)
  line L4 (0, 0) -> (0, -100)
  line L5 (0, -100) -> (79, -100)
  line L6 (79, -100) -> (79, 0)
  line L7 (79, 0) -> (0, 0)
  line L8 (63, -91) -> (75, -91)
  line L9 (75, -91) -> (75, -9)
  line L10 (75, -9) -> (63, -9)
  line L11 (63, -9) -> (63, -91)
  line L12 (39.6044, -92.1931) -> (39.6044, -7.1931)
  line L13 (4.2088, -9) -> (16.2088, -9)
  line L14 (4.2088, -91) -> (4.2088, -9)
  line L15 (16.2088, -9) -> (16.2088, -91)
  line L16 (16.2088, -91) -> (4.2088, -91)
  constraint horizontal L8
  constraint vertical L9
  constraint horizontal L10
  constraint vertical L11
  constraint midpoint L0 L12.start
  constraint midpoint L2 L12.end
  constraint symmetric L8.start L12 L15.end
  constraint symmetric L8.end L12 L14.start
  constraint symmetric L9.end L12 L13.start
  constraint symmetric L10.end L12 L13.end
extrude "Extrude12" cut sketch "Sketch8" against normal blind 30 contours L8 L9 L10 L11 | L13 L14 L15 L16 bodies 3
sketch "Sketch9" plane through (0, 0, -100) normal (0, 0, 1) x (1, 0, 0)
  line L0 (0, 7) -> (79, 7)
  line L1 (79, 7) -> (79, 24)
  line L2 (79, 24) -> (0, 24)
  line L3 (0, 24) -> (0, 7)
  line L4 (1, 23) -> (78, 23)
  line L5 (78, 23) -> (78, 22)
  line L6 (78, 22) -> (1, 22)
  line L7 (1, 22) -> (1, 23)
  line L8 (1, 21) -> (78, 21)
  line L9 (78, 21) -> (78, 20)
  line L10 (78, 20) -> (1, 20)
  line L11 (1, 20) -> (1, 21)
  line L12 (1, 19) -> (78, 19)
  line L13 (78, 19) -> (78, 18)
  line L14 (78, 18) -> (1, 18)
  line L15 (1, 18) -> (1, 19)
  constraint horizontal L4
  constraint vertical L5
  constraint horizontal L6
  constraint vertical L7
  constraint horizontal L8
  constraint vertical L9
  constraint horizontal L10
  constraint vertical L11
  constraint horizontal L12
  constraint vertical L13
  constraint horizontal L14
  constraint vertical L15
extrude "Extrude13" cut sketch "Sketch9" against normal blind 26 contours L4 L5 L6 L7 | L8 L9 L10 L11 | L12 L13 L14 L15 bodies 3
sketch "Sketch10" plane through (0, 0, 0) normal (1, 0, 0) x (0, 0, -1)
  line L0 (0, 7) -> (100, 7)
  line L1 (100, 7) -> (100, 24)
  line L2 (100, 24) -> (0, 24)
  line L3 (0, 24) -> (0, 7)
  line L4 (1, 23) -> (99, 23)
  line L5 (99, 23) -> (99, 22)
  line L6 (99, 22) -> (1, 22)
  line L7 (1, 22) -> (1, 23)
  line L8 (1, 21) -> (99, 21)
  line L9 (99, 21) -> (99, 20)
  line L10 (99, 20) -> (1, 20)
  line L11 (1, 20) -> (1, 21)
  line L12 (1, 19) -> (99, 19)
  line L13 (99, 19) -> (99, 18)
  line L14 (99, 18) -> (1, 18)
  line L15 (1, 18) -> (1, 19)
  constraint horizontal L4
  constraint vertical L5
  constraint horizontal L6
  constraint vertical L7
  constraint horizontal L8
  constraint vertical L9
  constraint horizontal L10
  constraint vertical L11
  constraint horizontal L12
  constraint vertical L13
  constraint horizontal L14
  constraint vertical L15
extrude "Extrude14" cut sketch "Sketch10" against normal blind 29 contours L4 L5 L6 L7 | L8 L9 L10 L11 | L12 L13 L14 L15 bodies 3
extrude "Extrude15" cut sketch "Sketch9" along normal blind 126 contours L4 L5 L6 L7 | L8 L9 L10 L11 | L12 L13 L14 L15 bodies 3
extrude "Extrude16" cut sketch "Sketch10" along normal blind 112 contours L4 L5 L6 L7 | L8 L9 L10 L11 | L12 L13 L14 L15 bodies 3
move_body "Move3" bodies 1 to x (1, 0, 0) y (0, 1, 0) z (0, 0, 1) at (0, 4, 0)
extrude "Extrude17" cut 1 faces at (32.5348, 24, -97.3977) along direction (0, 1, 0) blind 4 on bodies 3 bodies 3
sketch "Sketch11" plane through (0, 0, 0) normal (1, 0, 0) x (0, 0, -1)
  line L0 (99, 23) -> (99, 22)
  line L1 (99, 22) -> (1, 22)
  line L2 (1, 22) -> (1, 23)
  line L3 (1, 23) -> (99, 23)
  line L4 (99, 21) -> (99, 20)
  line L5 (99, 20) -> (1, 20)
  line L6 (1, 20) -> (1, 21)
  line L7 (1, 21) -> (99, 21)
  line L8 (99, 19) -> (99, 18)
  line L9 (99, 18) -> (1, 18)
  line L10 (1, 18) -> (1, 19)
  line L11 (1, 19) -> (99, 19)
  line L12 (0, 7) -> (100, 7)
  line L13 (100, 7) -> (100, 28)
  line L14 (100, 28) -> (0, 28)
  line L15 (0, 28) -> (0, 7)
  line L16 (0, 17.5) -> (0.65, 17.5)
  line L17 (100, 17.5) -> (99.35, 17.5)
  line L18 (0.6563, 28.6) -> (100, 28.6)
  line L19 (100, 28.6) -> (100, 8.6)
  line L20 (100, 8.6) -> (0.6563, 8.6)
  line L21 (0.6563, 8.6) -> (0.6563, 28.6)
  line L22 (99.35, 28.6) -> (99.35, 8.6)
  dimension "d46" = 0.65
  dimension "d47" = 0.65
  constraint midpoint L15 L16.start
  constraint perpendicular L10 L16
  constraint midpoint L13 L17.start
  constraint perpendicular L13 L17
  constraint horizontal L18
  constraint vertical L19
  constraint horizontal L20
  constraint vertical L21
  constraint coincident L13 L19.end
  constraint coincident L18 L22.start
  constraint coincident L20 L22.end
  constraint perpendicular L20 L22
  measures "d46" distance of L16.start L16.end
  measures "d47" distance of L17.start L17.end
extrude "Extrude18" cut 1 faces at (32.5348, 28, -97.3977) along direction (0, 1, 0) blind 1 on bodies 3 bodies 3
extrude "Extrude19" cut sketch "Sketch11" against normal blind 18 contours L14 L20 L21 L22 | L14 L18 L21 L22 bodies 3
sketch "Sketch12" plane through (0, 0, 0) normal (0, 1, 0) x (1, 0, 0)
  line L0 (0, 100) -> (80, 100)
  line L1 (80, 100) -> (80, 0)
  line L2 (80, 0) -> (0, 0)
  line L3 (0, 0) -> (0, 100)
  constraint horizontal L0
  constraint vertical L1
  constraint horizontal L2
  constraint vertical L3
move_body "Move4" bodies 3 to x (1, 0, 0) y (0, 1, 0) z (0, 0, 1) at (0, -5.5, 0)
extrude "Extrude20" add sketch "Sketch12" along normal blind 1.6 separate body makes body 4
sketch "Sketch13" plane through (0, -47.8659, -38.2927) normal (0, -0.780869, -0.624695) x (-1, 0, 0)
  line L0 (-1, 104.6364) -> (-1, 103.0356)
  line L1 (-1, 103.0356) -> (-78, 103.0356)
  line L2 (-78, 103.0356) -> (-78, 104.6364)
  line L3 (-78, 104.6364) -> (-100, 104.6364)
  line L4 (-100, 104.6364) -> (-79, 77.7433)
  line L5 (-79, 77.7433) -> (-79, 79.0239)
  line L6 (-79, 79.0239) -> (0, 79.0239)
  line L7 (0, 79.0239) -> (20, 104.6364)
  line L8 (20, 104.6364) -> (-1, 104.6364)
  line L9 (-78, 96.6325) -> (-78, 98.2333)
  line L10 (-78, 98.2333) -> (-1, 98.2333)
  line L11 (-1, 98.2333) -> (-1, 96.6325)
  line L12 (-1, 96.6325) -> (-78, 96.6325)
  line L13 (-78, 99.8341) -> (-78, 101.4349)
  line L14 (-78, 101.4349) -> (-1, 101.4349)
  line L15 (-1, 101.4349) -> (-1, 99.8341)
  line L16 (-1, 99.8341) -> (-78, 99.8341)
  line L17 (-80, 85) -> (0, 85)
  line L18 (0, 85) -> (0, 79.1)
  line L19 (0, 79.1) -> (-80, 79.1)
  line L20 (-80, 79.1) -> (-80, 85)
  constraint horizontal L17
  constraint vertical L18
  constraint horizontal L19
  constraint vertical L20
extrude "Extrude21" add sketch "Sketch13" along normal blind 5 contours L17 L18 L19 L20 bodies 3
sketch "Sketch14" plane through (0, 0.9146, -0.7317) normal (0, -0.780869, 0.624695) x (1, 0, 0)
  line L0 (78, 26.5495) -> (78, 24.9488)
  line L1 (78, 24.9488) -> (1, 24.9488)
  line L2 (1, 24.9488) -> (1, 26.5495)
  line L3 (1, 26.5495) -> (-20, 26.5495)
  line L4 (-20, 26.5495) -> (0, 0.937)
  line L5 (0, 0.937) -> (79, 0.937)
  line L6 (79, 0.937) -> (79, -0.3436)
  line L7 (79, -0.3436) -> (100, 26.5495)
  line L8 (100, 26.5495) -> (78, 26.5495)
  line L9 (1, 18.5456) -> (1, 20.1464)
  line L10 (1, 20.1464) -> (78, 20.1464)
  line L11 (78, 20.1464) -> (78, 18.5456)
  line L12 (78, 18.5456) -> (1, 18.5456)
  line L13 (1, 21.7472) -> (1, 23.348)
  line L14 (1, 23.348) -> (78, 23.348)
  line L15 (78, 23.348) -> (78, 21.7472)
  line L16 (78, 21.7472) -> (1, 21.7472)
  line L17 (0, 6.9105) -> (80, 6.9105)
  line L18 (80, 6.9105) -> (80, 1)
  line L19 (80, 1) -> (0, 1)
  line L20 (0, 1) -> (0, 6.9105)
  constraint horizontal L17
  constraint vertical L18
  constraint horizontal L19
  constraint vertical L20
extrude "Extrude22" add sketch "Sketch14" along normal blind 5 contours L17 L18 L19 L20 bodies 3
extrude "Extrude23" cut 1 faces at (26.6667, 1.0667, -100) along direction (0, 0, -1) blind 3 on bodies 4 bodies 3
extrude "Extrude24" cut 1 faces at (53.3333, 1.0667, 0) along direction (0, 0, 1) blind 3 on bodies 4 bodies 3
extrude "Extrude25" cut 1 faces at (26.6667, 0, -66.6667) along direction (0, 1, 0) blind 0.15 on bodies 4 bodies 4
extrude "Extrude26" cut 1 faces at (26.6667, 1.6, -66.6667) along direction (0, -1, 0) blind 0.1 on bodies 4 bodies 3 4
extrude "Extrude27" add 1 faces at (26.6667, 0.6, 0) along direction (0, 0, 1) blind 2.9 on bodies 4 bodies 3 4
extrude "Extrude28" add 1 faces at (53, 0.6, -100) along direction (0, 0, -1) blind 2.9 on bodies 3 bodies 3
extrude "Extrude29" add 1 faces at (53.3333, 0.1003, -106.2543) along direction (0, -0.780869, -0.624695) blind 5 on bodies 3 bodies 3
extrude "Extrude30" add 1 faces at (26.6667, 0.0965, 6.2495) along direction (0, -0.780869, 0.624695) blind 5 on bodies 3 bodies 3
extrude "Extrude31" cut 1 faces at (53.3333, 0.15, -67.6333) along direction (0, 1, 0) blind 1.4 on bodies 3 bodies 3
sketch "Sketch15" plane through (0, 1.6, 0) normal (0, -1, 0) x (1, 0, 0)
  line L0 (79, -100) -> (0, -100)
  line L1 (0, -100) -> (0, -100.125)
  line L2 (0, -100.125) -> (0, -103)
  line L3 (0, -103) -> (80, -103)
  line L4 (80, -103) -> (80, -100.125)
  line L5 (80, -100.125) -> (80, 0.125)
  line L6 (80, 0.125) -> (80, 3)
  line L7 (80, 3) -> (0, 3)
  line L8 (0, 3) -> (0, 0.125)
  line L9 (0, 0.125) -> (0, 0)
  line L10 (0, 0) -> (79, 0)
  line L11 (79, 0) -> (79, -100)
  line L12 (0.1, 2.9) -> (79.2, 2.9)
  line L13 (79.2, 2.9) -> (79.2, -102.9)
  line L14 (79.2, -102.9) -> (0.1, -102.9)
  line L15 (0.1, -102.9) -> (0.1, 2.9)
  constraint horizontal L12
  constraint vertical L13
  constraint horizontal L14
  constraint vertical L15
extrude "Extrude32" add sketch "Sketch15" along normal blind 1.5 separate body contours L0 L10 L11 L12 L13 L14 L15 | L0 L10 L11 L15 makes body 5
extrude "Extrude33" cut 1 faces at (52.8333, 1.6, -33.3333) along direction (0, -1, 0) blind 0.1 on bodies 5 bodies 5
sketch "Sketch16" plane through (0, 1.6, 0) normal (0, -1, 0) x (1, 0, 0)
  line L0 (79, -100) -> (0, -100)
  line L1 (0, -100) -> (0, -100.125)
  line L2 (0, -100.125) -> (0, -103)
  line L3 (0, -103) -> (80, -103)
  line L4 (80, -103) -> (80, -100.125)
  line L5 (80, -100.125) -> (80, 0.125)
  line L6 (80, 0.125) -> (80, 3)
  line L7 (80, 3) -> (0, 3)
  line L8 (0, 3) -> (0, 0.125)
  line L9 (0, 0.125) -> (0, 0)
  line L10 (0, 0) -> (79, 0)
  line L11 (79, 0) -> (79, -100)
  line L12 (80, 0.05) -> (79.4023, 0.05)
  line L13 (79.4023, 0.05) -> (79.4023, 3)
  line L14 (79.4023, 3) -> (80, 3)
  line L15 (80, 3) -> (80, 0.05)
  line L16 (79.4023, -100.05) -> (79.4023, -103)
  line L17 (80, -100.05) -> (79.4023, -100.05)
  line L18 (80, -103) -> (80, -100.05)
  line L19 (79.4023, -103) -> (80, -103)
  constraint horizontal L12
  constraint vertical L13
  constraint horizontal L14
  constraint vertical L15
  constraint coincident L7 L13.end
  constraint coincident L5 L12.start
extrude "Extrude34" add sketch "Sketch16" along normal blind 2 contours L3 L4 L5 L16 L17 L18 L19 | L5 L6 L7 L12 L13 L14 L15 bodies 3
hidden bodies 1 2 3
